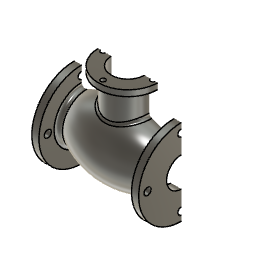
Flow Valve (Autodesk Fusion 360 design; units mm, degrees)
Autodesk Fusion 360 part; units mm, degrees
note: some values were not read from the file. Chosen so that the rebuilt part matches the saved one: which face or edge a step refers to.
sketch "Sketch1" plane through (0, 0, 0) normal (0, 1, 0) x (1, 0, 0)
  line L0 (-45, 0) -> (45, 0)
  line L1 (45, 0) -> (45, -36)
  line L2 (45, -36) -> (39, -36)
  line L3 (39, -36) -> (39, -18)
  line L4 (0, 0) -> (0, -54.0774) construction
  line L5 (-39, -36) -> (-39, -18)
  line L6 (-45, -36) -> (-39, -36)
  line L7 (-45, 0) -> (-45, -36)
  arc A0 (-39, -18) -> (39, -18) centre (0, 42.5227) ccw
  line L8 (-45, -12.5) -> (-36.2648, -12.5)
  line L9 (45, -12.5) -> (36.2648, -12.5)
  arc A1 (-36.2648, -12.5) -> (36.2648, -12.5) centre (0, 45.0227) ccw
  dimension "d1" = 90
  dimension "d2" = 36
  dimension "d3" = 18
  dimension "d4" = 72
  dimension "d5" = 6
  dimension "d6" = 68
  dimension "d7" = 12.5
  dimension "d8" = 2.5
  constraint horizontal L0
  constraint perpendicular L1 L2
  constraint perpendicular L2 L3
  constraint midpoint L4.start L0
  constraint coincident L4.start origin
  constraint perpendicular L0 L4
  constraint symmetric L0.end L4 L0.start
  constraint symmetric L1.end L4 L6.start
  constraint symmetric L2.end L4 L5.start
  constraint symmetric L3.end L4 L5.end
  constraint vertical L1
  constraint coincident L7 L8.start
  constraint perpendicular L7 L8
  constraint coincident L1 L9.start
  constraint perpendicular L1 L9
  constraint collinear L8 L9
  constraint vertical A0.centre A1.centre
  measures "d1" distance of L0.start L0.end
  measures "d2" distance of L0 L2
  measures "d3" distance of L0 L3.end
  measures "d4" radius of A0
  measures "d5" distance of L1.end L2.end
  measures "d6" radius of A1
  measures "d7" distance of L4.start L8
  measures "d8" distance of A0.centre A1.centre
revolve "Revolve1" add sketch "Sketch1" angle 360 about axis through (-45, 0, 0) along (1, 0, 0) contours L1 L2 L3 L5 L6 L7 A0 L8 L9 A1
ref_plane "WorkPlane1" through (0, 0, 55) normal (0, 0, 1) x (1, 0, 0)
sketch "Sketch2" plane through (0, 0, 55) normal (0, 0, 1) x (1, 0, 0)
  circle A0 centre (0, 0) radius 25
  circle A1 centre (0, 0) radius 18
  circle A2 centre (0, 0) radius 14
  dimension "d11" = 50
  dimension "d12" = 36
  dimension "d13" = 28
  constraint coincident A0.centre A1.centre
  constraint concentric A1 A2
  measures "d11" diameter of A0
  measures "d12" diameter of A1
  measures "d13" diameter of A2
extrude "Extrude1" add sketch "Sketch2" along normal up to surface contours A1 end surface at (-2.7469, 7.0418, 28.5698)
extrude "Extrude2" add sketch "Sketch2" against normal blind 5 contours A0
extrude "Extrude3" cut sketch "Sketch2" against normal blind 46 contours A2
sketch "Sketch3" plane through (0, 0, 0) normal (0, 1, 0) x (1, 0, 0)
  line L0 (-14, -5) -> (14, -5)
  line L1 (14, -5) -> (14, 5)
  line L2 (14, 5) -> (-14, 5)
  line L3 (-14, 5) -> (-14, -5)
  line L4 (14, -5) -> (29.8307, -16.0848)
  arc A0 (-36.2648, -12.5) -> (36.2648, -12.5) centre (0, 45.0227) ccw
  line L5 (14, -0.7273) -> (33.3193, -14.2548)
  arc A1 (29.8307, -16.0848) -> (33.3193, -14.2548) centre (0, 45.0227) ccw
  line L6 (-14, 5) -> (-29.8307, 16.0848)
  arc A2 (-29.8307, 16.0848) -> (-33.3193, 14.2548) centre (0, -45.0227) ccw
  line L7 (-14, 0.7273) -> (-33.3193, 14.2548)
  dimension "d20" = 28
  dimension "d21" = 10
  dimension "d22" = 5
  dimension "d23" = 14
  dimension "d24" = 145
  dimension "d27" = 360
  constraint horizontal L0
  constraint vertical L1
  constraint horizontal L2
  constraint vertical L3
  constraint coincident L4.end A0
  constraint coincident A0 L5.end
  constraint coincident L1 L5.start
  measures "d20" distance of L0.start L0.end
  measures "d21" distance of L0.start L2.end
  measures "d22" distance of origin L0
  measures "d23" distance of origin L1
  measures "d24" angle of L0 L4
extrude "Extrude4" add sketch "Sketch3" along normal mid plane 30
fillet "Fillet1" radius 2.5 6 edges at (-14, 0, 5) (14, 0, 5) (-14, 0, -0.7273) (14, 0, -5) (14, 0, 0.7273) (-14, 0, -5)
sketch "Sketch4" plane through (0, 0, 5) normal (0, 0, 1) x (-1, 0, 0)
  line L0 (-13.2118, 15) -> (-13.2118, -15)
  line L1 (-13.2118, -15) -> (11.5, -15)
  line L2 (11.5, -15) -> (11.5, 15)
  line L3 (11.5, 15) -> (-13.2118, 15)
  circle A0 centre (0, 0) radius 10
  dimension "d32" = 20
  constraint coincident A0.centre origin
  measures "d32" diameter of A0
extrude "Extrude5" cut sketch "Sketch4" against normal up to surface (10 mm away) draft -3 contours A0
chamfer "Chamfer1" distance 1 angle 45 2 edges at (9.3233, -3.6162, 5) (8.8347, 3.4266, -5)
fillet "Fillet2" radius 3 3 edges at (39, -6.5091, -16.7819) (-18.0001, -0.0115, 27.1907) (-39, -6.5091, -16.7819)
sketch "Sketch5" plane through (0, 0, 55) normal (0, 0, 1) x (-1, 0, 0)
  circle A0 centre (0, 0) radius 25
  circle A1 centre (0, 0) radius 14
  circle A2 centre (0, 0) radius 21 construction
  point P0 (0, -21)
  dimension "d38" = 42
  constraint concentric A0 A2
  constraint coincident A2 P0
  measures "d38" diameter of A2
hole "Hole1" at (0, 21, 55) direction (0, 0, -1) diameter 4 depth 18 tip angle 118
pattern_circular "C-Pattern1" count 4 over 360 about axis through (0, 0, 55) along (0, 0, -1) of "Hole1"
sketch "Sketch6" plane through (45, 0, 0) normal (1, 0, 0) x (0, 1, 0)
  circle A0 centre (0, 0) radius 12.5
  circle A1 centre (0, 0) radius 36
  circle A2 centre (0, 0) radius 28.5
  point P0 (0, -28.5)
  dimension "d44" = 57
  constraint coincident A0.centre A1.centre
  constraint coincident A2 P0
  measures "d44" diameter of A2
hole "Hole2" at (45, 0, -28.5) direction (-1, 0, 0) diameter 6 depth 7 tip angle 118
pattern_circular "C-Pattern2" count 4 over 360 about axis through (45, 0, 0) along (-1, 0, 0) of "Hole2"
mirror "Mirror1" about plane through (0, 0, 0) normal (1, 0, 0) of 4 faces at (41, 31.4851, 0.2987) (41, 0.2987, -31.4851) (41, -0.2987, 31.4851) (41, -31.4851, -0.2987)
equation "d23 = ( 28 / 2 ) * 1 mm"
